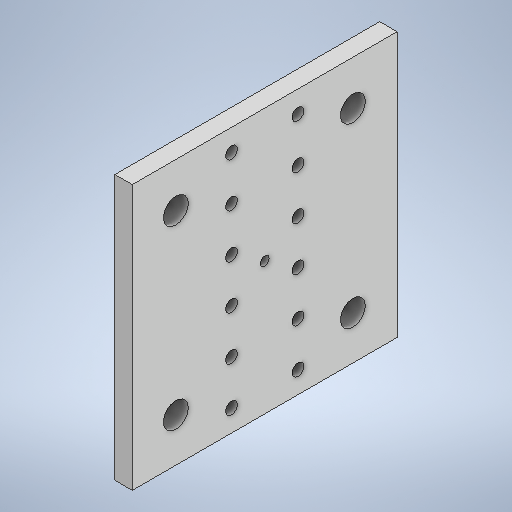
# Autodesk Inventor part: base_plate
Saved by Autodesk Inventor 2025 (Build 290162000, 162)
## iProperties
Created: 2025-12-10
Part Number: base_plate
Material: Generic
Document SubType Name: Modeling
Designer: GOLZARDM
Density: 1 g/cm^3
Appearance: Default
Author: GOLZARDM
Autodesk Inventor part; units mm, degrees
ref_plane "YZ Plane" through (0, 0, 0) normal (1, 0, 0) x (0, 1, 0)
ref_plane "XZ Plane" through (0, 0, 0) normal (0, 1, 0) x (-1, 0, 0)
ref_plane "XY Plane" through (0, 0, 0) normal (0, 0, 1) x (1, 0, 0)
sketch "Sketch5" plane through (0, 0, 0) normal (1, 0, 0) x (0, 1, 0)
  line L0 (76, -76) -> (-76, -76)
  line L1 (-76, -76) -> (-76, 76)
  line L2 (-76, 76) -> (76, 76)
  line L3 (76, 76) -> (76, -76)
  line L4 (76, -76) -> (-76, 76) construction
  line L5 (-76, -76) -> (76, 76) construction
  point P0 (0, 0)
  dimension "d31" = 152
  dimension "d32" = 152
  constraints: 12 end point, 2 midpoint, 2 parallel, 1 horizontal, 1 perpendicular
  measures "d31" distance of L2.end L0.start
  measures "d32" distance of L0.start L0.end
extrude "Extrusion2" add sketch "Sketch5" along normal blind 10
sketch "Sketch6" plane through (10, 0, 0) normal (1, 0, 0) x (0, 0, -1)
  line L0 (76, -76) -> (76, 76) projected
  line L1 (76, 76) -> (-76, 76) projected
  point P0 (0, 0)
  point P1 (50.6, 50.6)
  dimension "d42" = 25.4
  dimension "d43" = 25.4
  measures "d42" distance from line of L0 point (50.6, 50.6)
  measures "d43" distance from line of L1 point (50.6, 50.6)
hole "Hole4" at (10, 50.6, -50.6) direction (-1, 0, 0) diameter 14.3 end through all
sketch "Sketch7" plane through (10, 0, 0) normal (1, 0, 0) x (0, 0, -1)
  circle A0 centre (50.6, 50.6) radius 7.15 projected
  line L0 (76, 76) -> (-76, 76) projected
  point P0 (0, 0)
  point P1 (-51, 50.6)
  dimension "d51" = 101.6
  dimension "d52" = 25.4
  measures "d51" distance of A0.centre point (-51, 50.6)
  measures "d52" distance from line of L0 point (-51, 50.6)
hole "Hole5" at (10, 50.6, 51) direction (-1, 0, 0) diameter 14.3 end through all
sketch "Sketch8" plane through (10, 0, 0) normal (1, 0, 0) x (0, 0, -1)
  line L0 (76, -76) -> (76, 76) projected
  circle A0 centre (50.6, 50.6) radius 7.15 projected
  point P0 (0, 0)
  point P1 (50.6, -51)
  dimension "d60" = 25.4
  dimension "d61" = 101.6
  measures "d60" distance from line of L0 point (50.6, -51)
  measures "d61" distance of A0.centre point (50.6, -51)
hole "Hole6" at (10, -51, -50.6) direction (-1, 0, 0) diameter 14.3 end through all
sketch "Sketch9" plane through (10, 0, 0) normal (1, 0, 0) x (0, 0, -1)
  circle A0 centre (-51, 50.6) radius 7.15 projected
  circle A1 centre (50.6, -51) radius 7.15 projected
  point P0 (0, 0)
  point P1 (-51, -51)
  dimension "d69" = 101.6
  dimension "d70" = 101.6
  measures "d69" distance of A0.centre point (-51, -51)
  measures "d70" distance of point (-51, -51) A1.centre
hole "Hole7" at (10, -51, 51) direction (-1, 0, 0) diameter 14.3 end through all
sketch "Sketch10" plane through (10, 0, 0) normal (1, 0, 0) x (0, 0, -1)
  line L0 (76, 76) -> (-76, 76) projected
  line L1 (76, -76) -> (76, 76) projected
  point P0 (0, 0)
  point P1 (19.05, 63.5)
  dimension "d93" = 12.5
  dimension "d103" = 56.95
  measures "d93" distance from line of L0 point (19.05, 63.5)
  measures "d103" distance from line of L1 point (19.05, 63.5)
hole "Hole8" at (10, 63.5, -19.05) direction (-1, 0, 0) diameter 6.8 end through all
sketch "Sketch11" plane through (10, 0, 0) normal (1, 0, 0) x (0, 0, -1)
  circle A0 centre (19.05, 63.5) radius 3.4 projected
  point P0 (0, 0)
  point P1 (-19.05, 63.5)
  dimension "d85" = 38.1
  dimension "d86" = 0
  measures "d85" distance of A0.centre point (-19.05, 63.5)
  measures "d86" vertical distance of point (-19.05, 63.5) A0.centre
hole "Hole9" at (10, 63.5, 19.05) direction (-1, 0, 0) diameter 6.8 end through all
pattern_linear "Rectangular Pattern1" count 6 spacing 25.4 along (0, -1, 0) of "Hole8"
pattern_linear "Rectangular Pattern2" count 6 spacing 25.4 along (0, -1, 0) of "Hole9"
sketch "Sketch12" plane through (10, 0, 0) normal (1, 0, 0) x (0, 0, -1)
  line L0 (76, -76) -> (76, 76) projected
  line L1 (-76, -76) -> (76, -76) projected
  point P0 (0, 0)
  point P1 (0, 0)
  dimension "d101" = 76
  dimension "d102" = 76
  measures "d101" distance from line of L0 point (0, 0)
  measures "d102" distance from line of L1 point (0, 0)
hole "Hole10" at (10, 0, 0) direction (-1, 0, 0) diameter 5.2 end through all
body "Solid2"
